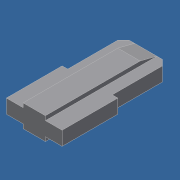
# Autodesk Inventor part: P1704_009_slider
Saved by Autodesk Inventor 2019 (Build 230136000, 136)
## iProperties
Created: 2019-05-02
Part Number: P1704_009_slider
Project: Nom Projet
Material: .
Description: Nom pièce
Document SubType Name: Modeling
Designer: Joan.MAILLARD
Authority: brut Ø
Density: 0.001 g/cm^3
Appearance: Par défaut
Author: Joan.MAILLARD
Material number: ---
Autodesk Inventor part; units mm, degrees
ref_plane "Plan YZ" through (0, 0, 0) normal (1, 0, 0) x (0, 1, 0)
ref_plane "Plan XZ" through (0, 0, 0) normal (0, 1, 0) x (-1, 0, 0)
ref_plane "Plan XY" through (0, 0, 0) normal (0, 0, 1) x (1, 0, 0)
sketch "Esquisse1" plane through (0, 0, 0) normal (0, 0, 1) x (1, 0, 0)
  line L0 (0, 0) -> (5, 0)
  line L1 (5, 0) -> (5, 5)
  line L2 (5, 5) -> (4.5, 5)
  line L3 (4.5, 5) -> (4.5, 10)
  line L4 (4.5, 10) -> (0.5, 10)
  line L5 (0.5, 10) -> (0.5, 5)
  line L6 (0.5, 5) -> (0, 5)
  line L7 (0, 5) -> (0, 0)
  dimension "d0" = 5
  dimension "d1" = 5
  dimension "d2" = 5
  dimension "d3" = 4
  constraints: 16 end point, 6 perpendicular, 2 point on line, 1 collinear, 1 horizontal
  measures "d0" distance of L0.start L0.end
  measures "d1" distance of L0.end L1.end
  measures "d2" distance of L2.end L3.end
  measures "d3" distance of L3.end L4.end
extrude "Extrusion1" add sketch "Esquisse1" along normal blind 1.25
sketch "Esquisse6" plane through (0, 0, 1.25) normal (0, 0, 1) x (1, 0, 0)
  line L0 (1.5, 0) -> (3.5, 0)
  line L1 (3.5, 0) -> (3.5, 10)
  line L2 (3.5, 10) -> (1.5, 10)
  line L3 (1.5, 10) -> (1.5, 0)
  line L4 (4.5, 10) -> (0.5, 10) projected
  line L5 (0, 0) -> (5, 0) projected
  line L6 (4.5, 5) -> (3.5, 5) construction
  line L7 (0.5, 5) -> (1.5, 5) construction
  dimension "d6" = 2
  constraints: 12 end point, 3 point on line, 2 midpoint, 2 parallel, 1 coincident, 1 collinear, 1 horizontal, 1 perpendicular
  measures "d6" distance of L1.end L2.end
extrude "Extrusion2" add sketch "Esquisse6" along normal blind 0.375 and the other way blind 1.625
sketch "Esquisse7" plane through (3.5, 0, 1.25) normal (1, 0, 0) x (0, 0, -1)
  line L0 (0, 10) -> (-0.375, 10)
  line L1 (-0.375, 10) -> (-0.375, 8.5)
  line L2 (-0.375, 8.5) -> (0, 10)
  line L3 (1.25, 10) -> (1.625, 8.5)
  line L4 (1.625, 8.5) -> (1.625, 10)
  line L5 (1.625, 10) -> (1.25, 10)
  point P0 (1.25, 0)
  dimension "d11" = 1.5
  dimension "d12" = 1.5
  constraints: 12 end point, 2 perpendicular, 1 coincident, 1 horizontal, 1 vertical
  measures "d11" distance of L0.end L1.end
  measures "d12" distance of L3.end L4.end
extrude "Extrusion3" cut sketch "Esquisse7" against normal blind 2
sketch "Esquisse8" plane through (0, 0, 0) normal (0, 0, -1) x (-1, 0, 0)
  line L0 (-4.5, 9.5) -> (-4, 10)
  line L1 (-4, 10) -> (-4.5, 10)
  line L2 (-4.5, 10) -> (-4.5, 9.5)
  line L3 (-1, 10) -> (-0.5, 9.5)
  line L4 (-0.5, 9.5) -> (-0.5, 10)
  line L5 (-0.5, 10) -> (-1, 10)
  point P0 (0, 0)
  point P1 (-0.5, 10)
  dimension "d15" = 0.5
  constraints: 12 end point, 3 equal length, 2 coincident, 2 perpendicular, 2 point on line, 1 horizontal, 1 parallel
  measures "d15" distance of L4.end L3.start
extrude "Extrusion4" cut sketch "Esquisse8" against normal blind 1.25
equation "\"d1\" = d0"
equation "\"d2\" = d1"
equation "\"d12\" = d11"
